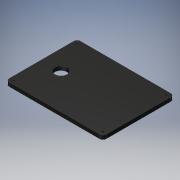
# Autodesk Inventor part: MainHousing_BottomPlate
Saved by Autodesk Inventor 2019 (Build 230136000, 136)
## iProperties
Created: 2018-09-02
Part Number: MainHousing_BottomPlate
Material: Generic
Document SubType Name: Modeling
Designer: Crater-Windows
Density: 1 g/cm^3
Appearance: Glossy - Black
Author: Crater-Windows
Autodesk Inventor part; units mm, degrees
ref_plane "YZ Plane" through (0, 0, 0) normal (1, 0, 0) x (0, 1, 0)
ref_plane "XZ Plane" through (0, 0, 0) normal (0, 1, 0) x (-1, 0, 0)
ref_plane "XY Plane" through (0, 0, 0) normal (0, 0, 1) x (1, 0, 0)
sketch "Sketch1" plane through (0, 0, 0) normal (0, 1, 0) x (-1, 0, 0)
  circle A0 centre (179.7843, -49) radius 2.65
  circle A1 centre (41.7843, 49) radius 2.65
  circle A2 centre (179.7843, 49) radius 2.65
  circle A3 centre (41.7843, -49) radius 2.65
  arc A4 (185.7843, 50) -> (180.7843, 55) centre (180.7843, 50) ccw
  line L0 (40.7843, 55) -> (180.7843, 55)
  arc A5 (40.7843, 55) -> (35.7843, 50) centre (40.7843, 50) ccw
  line L1 (35.7843, 12.5) -> (35.7843, 50)
  line L2 (35.7843, -50) -> (35.7843, -12.5)
  arc A6 (35.7843, -50) -> (40.7843, -55) centre (40.7843, -50) ccw
  line L3 (40.7843, -55) -> (180.7843, -55)
  arc A7 (180.7843, -55) -> (185.7843, -50) centre (180.7843, -50) ccw
  line L4 (185.7843, 50) -> (185.7843, -50)
  line L5 (35.7843, -12.5) -> (35.7843, 12.5)
  point P0 (0, 0)
  point P1 (35.7843, 55)
  constraints: 12 end point, 8 centre point, 8 point on circle, 4 vertical, 2 horizontal, 28 other
extrude "Extrusion1" add sketch "Sketch1" along normal blind 6
sketch "Sketch2" plane through (0, 6, 0) normal (0, 1, 0) x (1, 0, 0)
  circle A0 centre (-179.7843, 49) radius 2.65 projected
  circle A1 centre (-179.7843, 49) radius 1.65
  circle A2 centre (-41.7843, 49) radius 2.65 projected
  circle A3 centre (-41.7843, 49) radius 1.65
  circle A4 centre (-41.7843, -49) radius 2.65 projected
  circle A5 centre (-41.7843, -49) radius 1.65
  circle A6 centre (-179.7843, -49) radius 2.65 projected
  circle A7 centre (-179.7843, -49) radius 1.65
  point P0 (0, 0)
  dimension "d2" = 3.3
  dimension "d3" = 3.3
  dimension "d4" = 3.3
  dimension "d5" = 3.3
  constraints: 4 centre point, 4 coincident
  measures "d2" diameter of A1
  measures "d3" diameter of A3
  measures "d4" diameter of A5
  measures "d5" diameter of A7
extrude "Extrusion2" add sketch "Sketch2" against normal blind 6
sketch "Sketch3" plane through (0, 0, 0) normal (0, -1, 0) x (1, 0, 0)
  circle A0 centre (-155.7843, 0) radius 9.4
  line L0 (-185.7843, 50) -> (-185.7843, -50) projected
  line L1 (-40.7843, 55) -> (-180.7843, 55) projected
  point P0 (0, 0)
  dimension "d8" = 18.8
  dimension "d9" = 30
  dimension "d10" = 55
  constraints: 1 centre point
  measures "d8" diameter of A0
  measures "d9" distance from line of L0 A0.centre
  measures "d10" distance from line of A0.centre L1
extrude "Extrusion3" cut sketch "Sketch3" against normal blind 6
body "Solid1"
